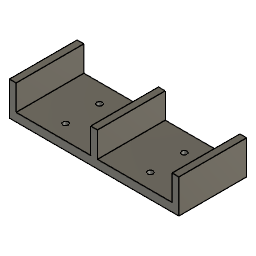
charging_dock_locator (Autodesk Fusion 360 design; units mm, degrees)
part number: 2026-06-07-21-21-21-460
Autodesk Fusion 360 part; units mm, degrees
sketch "Sketch1" plane through (0, 0, 0) normal (0, 0, 1) x (1, 0, 0)
  line L0 (-74.4245, 24.3877) -> (25.5755, 24.3877)
  line L1 (25.5755, 24.3877) -> (25.5755, -15.6123)
  line L2 (25.5755, -15.6123) -> (-74.4245, -15.6123)
  line L3 (-74.4245, -15.6123) -> (-74.4245, 24.3877)
  dimension "d1" = 100
  dimension "d2" = 40
  constraint horizontal L0
  constraint vertical L1
  constraint horizontal L2
  constraint vertical L3
  measures "d1" distance of L0.start L0.end
  measures "d2" distance of L0.start L2.end
extrude "Extrude1" add sketch "Sketch1" along normal blind 5
sketch "Sketch2" plane through (0, 0, 5) normal (0, 0, 1) x (-1, 0, 0)
  line L0 (74.4245, 15.6123) -> (-25.5755, 15.6123)
  line L1 (-25.5755, 15.6123) -> (-25.5755, -24.3877)
  line L2 (-25.5755, -24.3877) -> (74.4245, -24.3877)
  line L3 (74.4245, -24.3877) -> (74.4245, 15.6123)
  line L4 (74.4245, -24.3877) -> (70.4245, -24.3877)
  line L5 (70.4245, -24.3877) -> (70.4245, 15.6123)
  line L6 (70.4245, 15.6123) -> (74.4245, 15.6123)
  line L7 (74.4245, 15.6123) -> (74.4245, -24.3877)
  line L8 (-25.5755, -24.3877) -> (-21.5755, -24.3877)
  line L9 (-21.5755, -24.3877) -> (-21.5755, 15.6123)
  line L10 (-21.5755, 15.6123) -> (-25.5755, 15.6123)
  line L11 (-25.5755, 15.6123) -> (-25.5755, -24.3877)
  line L12 (26.4245, -24.3877) -> (22.4245, -24.3877)
  line L13 (22.4245, -24.3877) -> (22.4245, 15.6123)
  line L14 (22.4245, 15.6123) -> (26.4245, 15.6123)
  line L15 (26.4245, 15.6123) -> (26.4245, -24.3877)
  point P0 (24.4245, -24.3877)
  dimension "d5" = 4
  constraint horizontal L4
  constraint vertical L5
  constraint horizontal L6
  constraint vertical L7
  constraint coincident L0 L5.end
  constraint coincident L2.end L3.start
  constraint horizontal L8
  constraint vertical L9
  constraint horizontal L10
  constraint vertical L11
  constraint coincident L0 L9.end
  constraint coincident L1.end L2.start
  constraint horizontal L12
  constraint vertical L13
  constraint horizontal L14
  constraint vertical L15
  constraint coincident L0 L13.end
  constraint coincident L2 L12.start
  constraint coincident L2 P0
  constraint midpoint L2 P0
  constraint midpoint L12 P0
  constraint equal L6 L14
  constraint equal L10 L14
  measures "d5" distance of L5.end L0.start
extrude "Extrude2" add sketch "Sketch2" along normal blind 15 contours L0 L2 L3 L4 L5 L6 L7 | L0 L2 L12 L13 L14 L15 | L0 L1 L2 L8 L9 L10 L11
sketch "Sketch3" plane through (0, 0, 5) normal (0, 0, 1) x (-1, 0, 0)
  line L0 (26.4245, 15.6123) -> (26.4245, -24.3877)
  line L1 (26.4245, -24.3877) -> (70.4245, -24.3877)
  line L2 (70.4245, -24.3877) -> (70.4245, 15.6123)
  line L3 (70.4245, 15.6123) -> (26.4245, 15.6123)
  circle A0 centre (50.1716, -13.3243) radius 1.6
  circle A1 centre (50.1716, 6.6757) radius 1.6
  circle A2 centre (0.1716, -13.3243) radius 1.6
  circle A3 centre (0.1716, 6.6757) radius 1.6
  point P0 (0.1716, -13.3243)
  point P1 (50.1716, 6.6757)
  point P2 (0.1716, 6.6757)
  dimension "d8" = 3.2
  dimension "d11" = -50
  dimension "d12" = 20
  dimension "d15" = 3.2
  dimension "d16" = 3.2
  dimension "d17" = 3.2
  constraint coincident P1 A1.centre
  constraint coincident P0 A2.centre
  constraint coincident P2 A3.centre
  measures "d8" diameter of A0
  measures "d15" diameter of A1
  measures "d16" diameter of A2
  measures "d17" diameter of A3
extrude "Extrude3" cut sketch "Sketch3" against normal blind 5 contours A0 | A1 | A2 | A3
